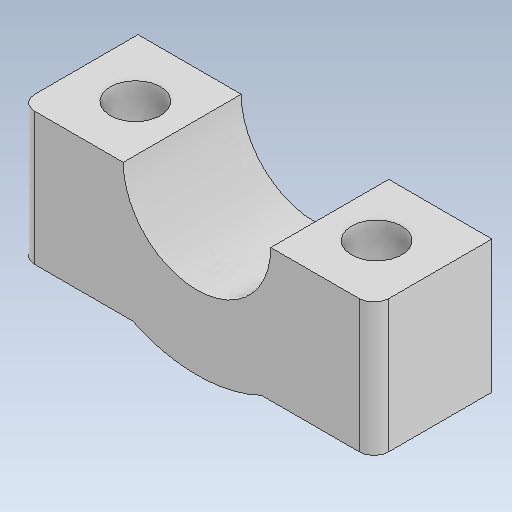
# Autodesk Inventor part: Bed Cable Harness Cable Clamp
Saved by Autodesk Inventor 2020 (Build 240168000, 168)
## iProperties
Created: 2019-12-21
Part Number: Bed Cable Harness Cable Clamp
Material: Generic
Document SubType Name: Modeling
Designer: pepd9
Density: 1 g/cm^3
Appearance: Default
Author: pepd9
Autodesk Inventor part; units mm, degrees
ref_plane "YZ Plane" through (0, 0, 0) normal (1, 0, 0) x (0, 1, 0)
ref_plane "XZ Plane" through (0, 0, 0) normal (0, 1, 0) x (-1, 0, 0)
ref_plane "XY Plane" through (0, 0, 0) normal (0, 0, 1) x (1, 0, 0)
sketch "Sketch1" plane through (0, 0, 0) normal (0, 0, 1) x (1, 0, 0)
  arc A0 (5, -5) -> (-5, -5) centre (0, -5) ccw projected
  circle A1 centre (0, -5) radius 5
  arc A2 (4.3589, 4) -> (-4.3589, 4) centre (0, -5) ccw projected
  line L0 (12, -5) -> (12, 4) projected
  line L1 (11, 4) -> (4.3589, 4) projected
  line L2 (12, 4) -> (0, 4)
  line L3 (0, 4) -> (0, -5)
  line L4 (0, -5) -> (12, -5)
  line L5 (12, -5) -> (12, 4)
  arc A3 (-4.3589, -14) -> (4.3589, -14) centre (0, -5) ccw
  line L6 (12, -5) -> (12, -14)
  line L7 (12, -14) -> (0, -14)
  line L8 (-12, -5) -> (-12, 4)
  line L9 (-12, 4) -> (0, 4)
  line L10 (0, -5) -> (-12, -5)
  line L11 (-12, -14) -> (0, -14)
  line L12 (-12, -5) -> (-12, -14)
  circle A4 centre (0, -5) radius 10
  point P0 (0, 0)
  constraints: 22 end point, 8 symmetric about line, 2 coincident, 2 parallel, 2 point on circle, 1 centre point, 1 horizontal, 1 perpendicular, 7 other
ref_plane "Work Plane1" through (-11, -5, -8) normal (0, 0, -1) x (0, 1, 0)
extrude "Extrusion1" add sketch "Sketch1" against normal up to surface (8 mm away) contours L4 A4 L7 L11 L10 A1 | L4 L6 L7 A4 | A4 L11 L12 L10 | A3 L11 L7
sketch "Sketch2" plane through (4.3589, -14, 0) normal (0, -1, 0) x (1, 0, 0)
  circle A0 centre (3.8206, -4) radius 1.7 projected
  circle A1 centre (-12.5383, -4) radius 1.7 projected
  point P0 (-4.3589, 0)
hole "Hole1" at (-8.1794, -14, -4) at (8.1794, -14, -4) direction (0, 1, 0) diameter 3.4 end through all counterbore diameter 6.5 counterbore depth 3 clearance for "Socket Head Cap Screw" size "M3" standard "Ansi Metric M Profile"
fillet "Fillet1" radius 1 2 edges at (12, -9.5, 0) (-12, -9.5, 0)
body "Solid1"
